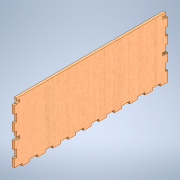
# Autodesk Inventor part: DoosjeRechterkant
Saved by Autodesk Inventor 2021 (Build 250183000, 183)
## iProperties
Created: 2021-03-11
Part Number: DoosjeRechterkant
Material: Wood (Cherry)
Document SubType Name: Modeling
Designer: ZiweZhang
Density: 0.63 g/cm^3
Appearance: Cherry - Natural Low Gloss
Author: ZiweZhang
Autodesk Inventor part; units mm, degrees
ref_plane "YZ Plane" through (0, 0, 0) normal (1, 0, 0) x (0, 1, 0)
ref_plane "XZ Plane" through (0, 0, 0) normal (0, 1, 0) x (-1, 0, 0)
ref_plane "XY Plane" through (0, 0, 0) normal (0, 0, 1) x (1, 0, 0)
sketch "Sketch1" plane through (0, 0, 0) normal (1, 0, 0) x (0, 1, 0)
  line L0 (0, 0) -> (77, 0)
  line L1 (77, 0) -> (77, -200)
  line L2 (77, -200) -> (0, -200)
  line L3 (0, -200) -> (0, 0)
  dimension "d0" = 77
  dimension "d1" = 200
  constraints: 8 end point, 2 parallel, 1 horizontal, 1 perpendicular
  measures "d0" distance of L1.end L2.end
  measures "d1" distance of L0.end L1.end
extrude "Extrusion1" add sketch "Sketch1" along normal blind 3
sketch "Sketch2" plane through (3, 0, 0) normal (1, 0, 0) x (0, 0, -1)
  line L0 (0, 77) -> (0, 0) projected
  line L1 (0, 0) -> (10, 0)
  line L2 (0, 0) -> (200, 0) projected
  line L3 (10, 0) -> (10, -3)
  line L4 (10, -3) -> (20, -3)
  line L5 (20, -3) -> (20, 0)
  line L6 (0, 0) -> (200, 0) projected
  line L7 (30, -3) -> (40, -3)
  line L8 (20, 0) -> (30, 0)
  line L9 (30, 0) -> (30, -3)
  line L10 (40, -3) -> (40, 0)
  line L11 (50, -3) -> (60, -3)
  line L12 (40, 0) -> (50, 0)
  line L13 (50, 0) -> (50, -3)
  line L14 (60, -3) -> (60, 0)
  line L15 (70, -3) -> (80, -3)
  line L16 (60, 0) -> (70, 0)
  line L17 (70, 0) -> (70, -3)
  line L18 (80, -3) -> (80, 0)
  line L19 (90, -3) -> (100, -3)
  line L20 (80, 0) -> (90, 0)
  line L21 (90, 0) -> (90, -3)
  line L22 (100, -3) -> (100, 0)
  line L23 (110, -3) -> (120, -3)
  line L24 (100, 0) -> (110, 0)
  line L25 (110, 0) -> (110, -3)
  line L26 (120, -3) -> (120, 0)
  line L27 (130, -3) -> (140, -3)
  line L28 (120, 0) -> (130, 0)
  line L29 (130, 0) -> (130, -3)
  line L30 (140, -3) -> (140, 0)
  line L31 (150, -3) -> (160, -3)
  line L32 (140, 0) -> (150, 0)
  line L33 (150, 0) -> (150, -3)
  line L34 (160, -3) -> (160, 0)
  line L35 (170, -3) -> (180, -3)
  line L36 (160, 0) -> (170, 0)
  line L37 (170, 0) -> (170, -3)
  line L38 (180, -3) -> (180, 0)
  line L39 (190, -3) -> (200, -3)
  line L40 (180, 0) -> (190, 0)
  line L41 (190, 0) -> (190, -3)
  line L42 (200, -3) -> (200, 0)
  line L43 (0, 0) -> (0, 10)
  line L44 (0, 10) -> (3, 10)
  line L45 (3, 10) -> (3, 20)
  line L46 (3, 20) -> (0, 20)
  line L47 (0, 20) -> (0, 30)
  line L48 (0, 30) -> (3, 30)
  line L49 (3, 30) -> (3, 40)
  line L50 (3, 40) -> (0, 40)
  line L51 (0, 40) -> (0, 50)
  line L52 (0, 50) -> (3, 50)
  line L53 (3, 50) -> (3, 60)
  line L54 (3, 60) -> (0, 60)
  line L55 (0, 60) -> (0, 70)
  line L56 (0, 70) -> (3, 70)
  line L57 (3, 70) -> (3, 77)
  line L58 (200, 77) -> (0, 77) projected
  line L59 (200, 0) -> (200, 77) projected
  line L60 (200, 0) -> (200, 10)
  line L61 (197, 10) -> (197, 20)
  line L62 (197, 20) -> (200, 20)
  line L63 (200, 30) -> (197, 30)
  line L64 (197, 30) -> (197, 40)
  line L65 (197, 40) -> (200, 40)
  line L66 (200, 40) -> (200, 50)
  line L67 (200, 50) -> (197, 50)
  line L68 (197, 50) -> (197, 60)
  line L69 (197, 60) -> (200, 60)
  line L70 (200, 60) -> (200, 70)
  line L71 (200, 70) -> (197, 70)
  line L72 (197, 70) -> (197, 77)
  line L73 (200, 10) -> (197, 10)
  line L74 (200, 20) -> (200, 30)
  line L75 (3, 77) -> (197, 77)
  dimension "d4" = 10
  dimension "d9" = 20
  dimension "d14" = 10
  dimension "d15" = 3
  dimension "d16" = 10
  dimension "d19" = 20
  dimension "d24" = 10
  dimension "d25" = 10
  constraints: 142 end point, 20 point on line, 13 perpendicular, 2 collinear, 2 horizontal, 2 vertical, 1 parallel, 99 other
  measures "d4" distance of L0.end L1.end
  measures "d9" distance of L3.end L7.start
  measures "d14" distance of L0.end L43.end
  measures "d15" distance of L43.end L44.end
  measures "d16" distance of L44.end L45.end
  measures "d19" distance of L0.end L47.start
  measures "d24" distance of L54.end L55.end
  measures "d25" distance of L61.start L61.end
extrude "Extrusion2" cut sketch "Sketch2" against normal blind 3 contours L56 L57 L58 L72 L71 L59 L69 L68 L67 L65 L64 L63 L62 L61 L73 L2 L1 L0 L44 L45 L46 L48 L49 L50 L52 L53 L54 keep common part
sketch "Sketch3" plane through (3, 0, 0) normal (1, 0, 0) x (0, 0, -1)
  line L0 (0, 0) -> (10, 0)
  line L1 (0, 0) -> (200, 0)
  line L2 (10, 0) -> (10, -3)
  line L3 (10, -3) -> (20, -3)
  line L4 (20, -3) -> (20, 0)
  line L5 (30, -3) -> (40, -3)
  line L6 (20, 0) -> (30, 0)
  line L7 (30, 0) -> (30, -3)
  line L8 (40, -3) -> (40, 0)
  line L9 (50, -3) -> (60, -3)
  line L10 (40, 0) -> (50, 0)
  line L11 (50, 0) -> (50, -3)
  line L12 (60, -3) -> (60, 0)
  line L13 (70, -3) -> (80, -3)
  line L14 (60, 0) -> (70, 0)
  line L15 (70, 0) -> (70, -3)
  line L16 (80, -3) -> (80, 0)
  line L17 (90, -3) -> (100, -3)
  line L18 (80, 0) -> (90, 0)
  line L19 (90, 0) -> (90, -3)
  line L20 (100, -3) -> (100, 0)
  line L21 (110, -3) -> (120, -3)
  line L22 (100, 0) -> (110, 0)
  line L23 (110, 0) -> (110, -3)
  line L24 (120, -3) -> (120, 0)
  line L25 (130, -3) -> (140, -3)
  line L26 (120, 0) -> (130, 0)
  line L27 (130, 0) -> (130, -3)
  line L28 (140, -3) -> (140, 0)
  line L29 (150, -3) -> (160, -3)
  line L30 (140, 0) -> (150, 0)
  line L31 (150, 0) -> (150, -3)
  line L32 (160, -3) -> (160, 0)
  line L33 (170, -3) -> (180, -3)
  line L34 (160, 0) -> (170, 0)
  line L35 (170, 0) -> (170, -3)
  line L36 (180, -3) -> (180, 0)
  line L37 (190, -3) -> (200, -3)
  line L38 (180, 0) -> (190, 0)
  line L39 (190, 0) -> (190, -3)
  line L40 (10, 0) -> (10, -3)
  line L41 (20, -3) -> (20, 0)
  line L42 (0, 0) -> (30, 0)
  line L43 (40, 0) -> (200, 0)
  line L44 (0, 0) -> (200, 0) projected
  line L45 (200, -3) -> (200, 0)
  dimension "d28" = 10
  dimension "d29" = 3
  dimension "d30" = 10
  dimension "d31" = 20
  constraints: 88 end point, 3 perpendicular, 1 collinear, 1 point on line, 1 vertical, 5 other
  measures "d28" distance of L0.start L0.end
  measures "d29" distance of L0.end L2.end
  measures "d30" distance of L2.end L4.start
  measures "d31" distance of L2.end L7.end
extrude "Extrusion3" add sketch "Sketch3" against normal blind 3
sketch "Sketch4" plane through (3, 0, 0) normal (1, 0, 0) x (0, 0, -1)
  line L0 (197, 70) -> (197, 77) projected
  line L1 (197, 74) -> (193, 74)
  line L2 (193, 74) -> (193, 71)
  line L3 (193, 71) -> (197, 71)
  line L4 (197, 71) -> (197, 74)
  line L5 (7, 74) -> (3, 74)
  line L6 (3, 74) -> (3, 71)
  line L7 (3, 71) -> (7, 71)
  line L8 (7, 71) -> (7, 74)
  line L9 (197, 33) -> (193, 33)
  line L10 (193, 33) -> (193, 30)
  line L11 (193, 30) -> (197, 30)
  line L12 (197, 30) -> (197, 33)
  line L13 (7, 33) -> (3, 33)
  line L14 (3, 33) -> (3, 30)
  line L15 (3, 30) -> (7, 30)
  line L16 (7, 30) -> (7, 33)
  point P0 (0, 0)
  dimension "d34" = 4
  dimension "d35" = 3
  dimension "d38" = 190
  dimension "d41" = 41
  constraints: 32 end point, 2 collinear, 2 horizontal, 2 parallel, 1 perpendicular, 1 point on line, 1 vertical, 22 other
  measures "d34" distance of L3.end L2.end
  measures "d35" distance of L2.end L1.end
  measures "d38" distance of L1.start L5.start
  measures "d41" distance of L1.start L9.start
extrude "Extrusion4" cut sketch "Sketch4" against normal through all
body "Solid1"
